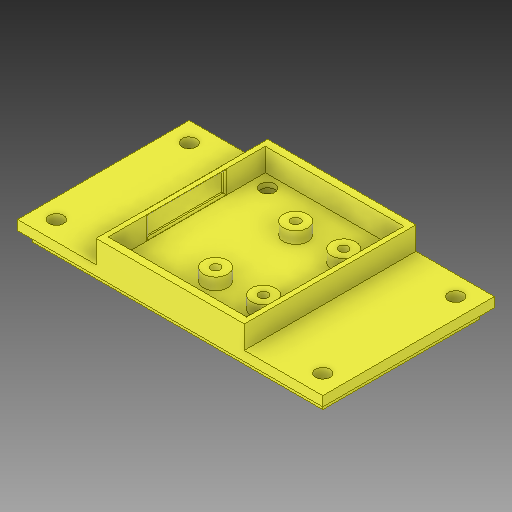
# Autodesk Inventor part: CaseTopForPiZeroWandCamera
Saved by Autodesk Inventor 2019.3 (Build 233278000, 278)
## iProperties
Created: 2018-12-18
Part Number: CaseTopForPiZeroWandCamera
Material: Polypropylene
Document SubType Name: Modeling
Designer: steele
Density: 0.899 g/cm^3
Appearance: Smooth - Yellow
Author: steele
Autodesk Inventor part; units mm, degrees
ref_plane "YZ Plane" through (0, 0, 0) normal (1, 0, 0) x (0, 1, 0)
ref_plane "XZ Plane" through (0, 0, 0) normal (0, 1, 0) x (-1, 0, 0)
ref_plane "XY Plane" through (0, 0, 0) normal (0, 0, 1) x (1, 0, 0)
sketch "Sketch1" plane through (0, 0, 0) normal (0, 1, 0) x (-1, 0, 0)
  line L0 (40, 22.5) -> (-40, 22.5)
  line L1 (-40, 22.5) -> (-40, -22.5)
  line L2 (-40, -22.5) -> (40, -22.5)
  line L3 (40, -22.5) -> (40, 22.5)
  line L4 (40, 22.5) -> (-40, -22.5) construction
  line L5 (-40, 22.5) -> (40, -22.5) construction
  point P0 (0, 0)
  dimension "d0" = 80
  dimension "d1" = 45
  constraints: 12 end point, 2 midpoint, 2 parallel, 1 horizontal, 1 perpendicular
  measures "d0" distance of L0.start L0.end
  measures "d1" distance of L2.end L0.start
extrude "ExtrusionForTopOfCase" add sketch "Sketch1" against normal blind 2.54
sketch "Sketch2" plane through (0, -2.54, 0) normal (0, -1, 0) x (1, 0, 0)
  line L0 (40, 22.5) -> (-40, 22.5) projected
  line L1 (-40, 22.5) -> (-40, -22.5) projected
  line L2 (40, 22.5) -> (-40, 22.5)
  line L3 (-40, 22.5) -> (-40, -22.5)
  line L4 (-40, -22.5) -> (40, -22.5)
  line L5 (40, -22.5) -> (40, 22.5)
  line L6 (38.095, 20.595) -> (-38.095, 20.595)
  line L7 (-38.095, 20.595) -> (-38.095, -20.595)
  line L8 (-38.095, -20.595) -> (38.095, -20.595)
  line L9 (38.095, -20.595) -> (38.095, 20.595)
  line L10 (38.095, 20.595) -> (-38.095, -20.595) construction
  line L11 (-38.095, 20.595) -> (38.095, -20.595) construction
  point P0 (0, 0)
  dimension "d6" = 1.905
  dimension "d7" = 1.905
  constraints: 20 end point, 4 parallel, 2 horizontal, 2 midpoint, 2 perpendicular
  measures "d6" distance between parallel lines of L6 L0
  measures "d7" distance between parallel lines of L5 L9
extrude "ExtrusionForBottomRidge" add sketch "Sketch2" along normal blind 2.54 contours L9 L8 L7 L6
sketch "Sketch8" plane through (0, 0, 0) normal (0, 1, 0) x (1, 0, 0)
  line L0 (-34.92, -17.42) -> (34.92, -17.42) construction
  line L1 (34.92, -17.42) -> (34.92, 17.42) construction
  line L2 (34.92, 17.42) -> (-34.92, 17.42) construction
  line L3 (-34.92, 17.42) -> (-34.92, -17.42) construction
  line L4 (38.095, 20.595) -> (-38.095, 20.595) construction
  line L5 (-38.095, 20.595) -> (-38.095, -20.595) construction
  line L6 (-38.095, -20.595) -> (38.095, -20.595) construction
  line L7 (38.095, -20.595) -> (38.095, 20.595) construction
  point P0 (0, 0)
  dimension "d39" = 3.175
  dimension "d40" = 3.175
  dimension "d41" = 3.175
  dimension "d42" = 3.175
  constraints: 8 end point, 4 coincident, 2 parallel, 1 horizontal, 1 perpendicular
  measures "d39" distance between parallel lines of L2 L4
  measures "d40" distance between parallel lines of L5 L3
  measures "d41" distance between parallel lines of L6 L0
  measures "d42" distance between parallel lines of L7 L1
sketch "Sketch11" plane through (0, 0, 0) normal (0, 1, 0) x (1, 0, 0)
  line L0 (40, -22.5) -> (-40, -22.5) projected
  line L1 (-40, 22.5) -> (40, 22.5) projected
  line L2 (-19.426, -22.5) -> (19.436, -22.5)
  line L3 (19.436, -22.5) -> (19.436, 22.5)
  line L4 (19.436, 22.5) -> (-19.426, 22.5)
  line L5 (-19.426, 22.5) -> (-19.426, -22.5)
  line L6 (-40, 22.5) -> (-40, -22.5) projected
  line L7 (-38.095, -20.595) -> (38.095, -20.595) projected
  line L8 (-38.095, 20.595) -> (38.095, 20.595) projected
  line L9 (-18.156, -20.595) -> (18.166, -20.595)
  line L10 (18.166, -20.595) -> (18.166, 20.595)
  line L11 (18.166, 20.595) -> (-18.156, 20.595)
  line L12 (-18.156, 20.595) -> (-18.156, -20.595)
  point P0 (0, 0)
  dimension "d57" = 20.574
  dimension "d58" = 1.27
  dimension "d59" = 1.27
  dimension "d60" = 59.436
  constraints: 16 end point, 4 parallel, 4 point on line, 2 horizontal, 2 perpendicular
  measures "d57" distance between parallel lines of L5 L6
  measures "d58" distance between parallel lines of L5 L12
  measures "d59" distance between parallel lines of L3 L10
  measures "d60" distance between parallel lines of L3 L6
extrude "Extrusion7" add sketch "Sketch11" along normal blind 6 contours L0 L5 L7 L3 | L7 L10 L8 L3 | L5 L8 L12 L7 | L8 L5 L1 L3
sketch "Sketch13" plane through (-19.426, 0, -22.5) normal (-1, 0, 0) x (0, 0, 1)
  line L0 (43.095, 6) -> (1.905, 6) construction
  line L1 (22.5, 6) -> (22.5, 0) construction
  line L2 (12.5, 0.5) -> (32.5, 0.5)
  line L3 (32.5, 0.5) -> (32.5, 5.5)
  line L4 (32.5, 5.5) -> (12.5, 5.5)
  line L5 (12.5, 5.5) -> (12.5, 0.5)
  line L6 (12.5, 0.5) -> (32.5, 5.5) construction
  line L7 (32.5, 0.5) -> (12.5, 5.5) construction
  line L8 (0, 6) -> (45, 6) projected
  point P0 (22.5, 3)
  dimension "d70" = 5
  dimension "d71" = 20
  constraints: 14 end point, 4 midpoint, 3 parallel, 1 perpendicular, 1 vertical
  measures "d70" distance of L4.end L2.start
  measures "d71" distance of L3.end L4.end
extrude "Extrusion8" cut sketch "Sketch13" against normal up to next
fillet "Fillet1" radius 0.4233 8 edges at (-18.156, 0.5, 0) (-18.156, 3, 10) (-18.156, 5.5, 0) (-18.156, 3, -10) (-19.426, 0.5, 0) (-19.426, 5.5, 0) (-19.426, 3, 10) (-19.426, 3, -10)
hole "Hole7" at (-34.92, 0, -17.42) at (34.92, 0, -17.42) at (34.92, 0, 17.42) at (-34.92, 0, 17.42) direction (0, -1, 0) diameter 3.81 end through all clearance for "Flat Head Machine Screw (82)" size "#6" standard "Ansi Unified Screw Threads"
sketch "Sketch21" plane through (0, -5.08, 0) normal (0, -1, 0) x (1, 0, 0)
  circle A0 centre (34.92, 17.42) radius 1.905 projected
  circle A1 centre (-34.92, -17.42) radius 1.905 projected
  circle A2 centre (34.92, -17.42) radius 1.905 projected
  circle A3 centre (-34.92, 17.42) radius 1.905 projected
  line L0 (38.095, 20.595) -> (-38.095, 20.595) projected
  line L1 (-38.095, 20.595) -> (-38.095, -20.595) projected
  line L2 (-38.095, -20.595) -> (38.095, -20.595) projected
  line L3 (38.095, -20.595) -> (38.095, 20.595) projected
  circle A4 centre (-14.346, 17.42) radius 1.2657 projected
  circle A5 centre (14.356, 17.42) radius 1.2657 projected
  circle A6 centre (14.356, -17.42) radius 1.2657 projected
  circle A7 centre (-14.346, -17.42) radius 1.2657 projected
  point P0 (0, 0)
  constraints: 4 coincident
hole "Hole12" at (-14.346, -5.08, 17.42) at (14.356, -5.08, 17.42) at (14.356, -5.08, -17.42) at (-14.346, -5.08, -17.42) direction (0, 1, 0) diameter 3.8354 end through all counterbore diameter 4.8514 counterbore depth 3.81
sketch "Sketch22" plane through (0, 0, 0) normal (0, 1, 0) x (1, 0, 0)
  line L0 (40, -22.5) -> (40, 22.5) projected
  line L1 (19.436, -22.5) -> (40, -22.5) projected
  circle A0 centre (12.48, 10.5) radius 3.175
  circle A1 centre (12.48, -10.5) radius 3.175
  circle A2 centre (-0.1, -10.5) radius 3.175
  circle A3 centre (-0.1, 10.5) radius 3.175
  point P0 (0, 0)
  dimension "d130" = 27.52
  dimension "d131" = 12
  dimension "d132" = 12.58
  dimension "d133" = 21
  dimension "d134" = 12.58
  dimension "d135" = 21
  dimension "d136" = 6.35
  constraints: 4 centre point, 4 coincident, 3 equal radius
  measures "d130" distance from line of L0 point (12.48, -10.5)
  measures "d131" distance from line of L1 point (12.48, -10.5)
  measures "d132" distance of point (-0.1, -10.5) point (12.48, -10.5)
  measures "d133" distance of point (12.48, 10.5) point (12.48, -10.5)
  measures "d134" distance of point (-0.1, 10.5) point (12.48, 10.5)
  measures "d135" distance of point (-0.1, -10.5) point (-0.1, 10.5)
  measures "d136" diameter of A0
extrude "Extrusion10" add sketch "Sketch22" along normal blind 3.1
sketch "Sketch24" plane through (0, -5.08, 0) normal (0, -1, 0) x (1, 0, 0)
  circle A0 centre (-0.1, -10.5) radius 3.175 projected
  circle A1 centre (12.48, -10.5) radius 3.175 projected
  circle A2 centre (12.48, 10.5) radius 3.175 projected
  circle A3 centre (-0.1, 10.5) radius 3.175 projected
  circle A4 centre (-0.1, -10.5) radius 3.175 projected
  point P0 (0, 0)
  constraints: 4 coincident
hole "Hole14" at (-0.1, -5.08, -10.5) at (-0.1, -5.08, 10.5) at (12.48, -5.08, 10.5) at (12.48, -5.08, -10.5) direction (0, 1, 0) diameter 2.4384 end through all counterbore diameter 3.2639 counterbore depth 3.9878
equation "\"d0\" = CaseLength"
equation "\"d1\" = CaseWidth"
equation "\"d2\" = TopExtensionHeight"
equation "\"d8\" = LowerExtenstionHeight"
equation "\"d58\" = CaseWallThickness"
equation "\"d59\" = CaseWallThickness"
equation "\"d70\" = PiRibbonCableThickness"
equation "\"d71\" = PiRibbonCableWidth"
equation "\"d74\" = FilletForRibbonCable"
equation "\"TopTotalHeight\" = 5.08"
equation "\"TopExtensionHeight\" = 0.5 * TopTotalHeight"
equation "\"LowerExtenstionHeight\" = 0.5 * TopTotalHeight"
equation "\"CaseLength\" = 80"
equation "\"CaseWidth\" = 45"
equation "\"CaseWallThickness\" = 1.27"
equation "\"PiRibbonCableThickness\" = 5"
equation "\"PiRibbonCableWidth\" = 20"
equation "\"FilletForRibbonCable\" = 0.423333"
body "Solid1"
